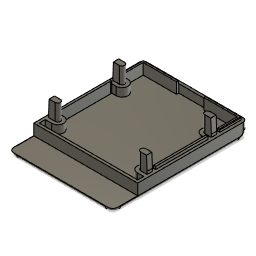
Ensoniq Cartridge Case EEPROM v32 (Autodesk Fusion 360 design; units mm, degrees)
Autodesk Fusion 360 part; units mm, degrees
note: some values were not read from the file. Set by a fixed rule: which face or edge a step refers to.
sketch "Sketch1" plane through (0, 0, 0) normal (0, 1, 0) x (1, 0, 0) in component "PCB"
  line L0 (19.8437, -28.575) -> (-19.8437, -28.575)
  line L1 (-19.8437, -28.575) -> (-19.8437, 28.575)
  line L2 (-19.8437, 28.575) -> (19.8438, 28.575)
  line L3 (19.8438, 28.575) -> (19.8437, -28.575)
  line L4 (19.8437, -28.575) -> (-19.8437, 28.575) construction
  line L5 (-19.8437, -28.575) -> (19.8438, 28.575) construction
  circle A0 centre (-19.8437, 20.32) radius 1.5
  circle A1 centre (-19.8437, -9.525) radius 1.5
  circle A2 centre (19.8438, 20.32) radius 1.5
  circle A3 centre (19.8437, -9.525) radius 1.5
  circle A4 centre (-19.8437, 20.32) radius 1.246
  circle A5 centre (19.8438, 20.32) radius 1.246
  circle A6 centre (19.8437, -9.525) radius 1.246
  circle A7 centre (-19.8437, -9.525) radius 1.246
  dimension "d1" = 57.15
  dimension "d2" = 39.6875
  dimension "d3" = 3
  dimension "d4" = 3
  dimension "d5" = 3
  dimension "d6" = 3
  dimension "d7" = 19.05
  dimension "d8" = 29.845
  dimension "d40" = -0.254
  dimension "d41" = -0.254
  dimension "d42" = -0.254
  dimension "d43" = -0.254
  constraint horizontal L0
  constraint perpendicular L0 L1
  constraint parallel L0 L2
  constraint parallel L1 L3
  constraint coincident L4 origin
  constraint coincident L5 origin
  constraint coincident L1 A0.centre
  constraint coincident L1 A1.centre
  constraint coincident L3 A2.centre
  constraint coincident L3 A3.centre
  constraint horizontal A1.centre A3.centre
  constraint horizontal A0.centre A2.centre
  measures "d1" distance of L0.end L1.end
  measures "d2" distance of L1.end L2.end
  measures "d3" diameter of A0
  measures "d4" diameter of A1
  measures "d5" diameter of A2
  measures "d6" diameter of A3
  measures "d7" distance of L0.end A1.centre
  measures "d8" distance of A0.centre A1.centre
extrude "Extrude1" add sketch "Sketch1" along normal blind 1.6 contours L0 L1 L2 L3 A0 A1 A2 A3 makes body 1 in component "PCB"
sketch "Sketch1 (2)" plane through (0, 0, 0) normal (0, 1, 0) x (1, 0, 0) in component "Back"
  line L0 (19.8438, 18.82) -> (19.8437, -8.025) construction
  arc A0 (19.8437, -8.025) -> (19.8437, -11.025) centre (19.8437, -9.525) ccw construction
  line L1 (19.8437, -11.025) -> (19.8437, -28.575) construction
  line L2 (19.8437, -28.575) -> (-19.8437, -28.575) construction
  line L3 (-19.8437, -28.575) -> (-19.8437, -11.025) construction
  arc A1 (-19.8437, -11.025) -> (-19.8437, -8.025) centre (-19.8437, -9.525) ccw construction
  line L4 (-19.8437, -8.025) -> (-19.8437, 18.82) construction
  arc A2 (-19.8437, 18.82) -> (-19.8437, 21.82) centre (-19.8437, 20.32) ccw construction
  line L5 (-19.8437, 21.82) -> (-19.8438, 28.575) construction
  line L6 (-19.8437, 28.575) -> (19.8438, 28.575) construction
  line L7 (19.8438, 28.575) -> (19.8438, 21.82) construction
  arc A3 (19.8438, 21.82) -> (19.8437, 18.82) centre (19.8438, 20.32) ccw construction
  line L8 (24.13, -16.383) -> (-24.13, -16.383)
  line L9 (-24.13, -16.383) -> (-24.13, 34.417)
  line L10 (-24.13, 34.417) -> (24.13, 34.417)
  line L11 (24.13, 34.417) -> (24.13, -16.383)
  line L12 (24.13, -16.383) -> (-24.13, 34.417) construction
  line L13 (-24.13, -16.383) -> (24.13, 34.417) construction
  line L14 (22.86, 33.147) -> (22.86, -15.113)
  line L15 (22.86, -15.113) -> (-22.86, -15.113)
  line L16 (-22.86, -15.113) -> (-22.86, 33.147)
  line L17 (-22.86, 33.147) -> (22.86, 33.147)
  point P0 (0, 9.017)
  dimension "d11" = 48.26
  dimension "d12" = 50.8
  dimension "d13" = 12.192
  dimension "d14" = 1.27
  constraint horizontal L8
  constraint perpendicular L8 L9
  constraint parallel L8 L10
  constraint parallel L9 L11
  constraint coincident L12 P0
  constraint coincident L13 P0
  constraint vertical origin P0
  measures "d11" distance of L9.end L10.end
  measures "d12" distance of L8.end L9.end
  measures "d13" distance of L2 L8
extrude "Extrude1'" add sketch "Sketch1 (2)" against normal blind 5.08 separate body contours L8 L9 L10 L11 | L14 L15 L16 L17 makes body 2 in component "Back"
sketch "Sketch1 (3)" plane through (0, 0, 0) normal (0, 1, 0) x (1, 0, 0) in component "Front"
  line L0 (-24.13, -16.383) -> (-24.13, 34.417)
  line L1 (24.13, -16.383) -> (-24.13, -16.383)
  line L2 (24.13, 34.417) -> (24.13, -16.383)
  line L3 (-24.13, 34.417) -> (24.13, 34.417)
extrude "Extrude1''" add sketch "Sketch1 (3)" along normal blind 6.604 separate body makes body 3 in component "Front"
sketch "Sketch2" plane through (0, 6.604, 0) normal (0, 1, 0) x (-1, 0, 0) in component "Front"
  line L0 (24.13, -34.417) -> (24.13, 16.383)
  line L1 (24.13, 16.383) -> (-24.13, 16.383)
  line L2 (-24.13, 16.383) -> (-24.13, -34.417)
  line L3 (-24.13, -34.417) -> (24.13, -34.417)
  line L4 (24.13, -34.417) -> (-24.13, -34.417)
  line L5 (-24.13, -34.417) -> (-24.13, 16.383)
  line L6 (-24.13, 16.383) -> (24.13, 16.383)
  line L7 (24.13, 16.383) -> (24.13, -34.417)
  line L8 (24.13, 16.383) -> (-24.13, 16.383)
  line L9 (-24.13, 16.383) -> (-24.13, 27.94)
  line L10 (-24.13, 27.94) -> (24.13, 27.94)
  line L11 (24.13, 27.94) -> (24.13, 16.383)
  dimension "d19" = 11.557
  constraint horizontal L8
  constraint vertical L9
  constraint horizontal L10
  constraint vertical L11
  constraint coincident L0.end L1.start
  measures "d19" distance of L0.end L10.end
extrude "Extrude2" add sketch "Sketch2" along normal blind 5.08 bodies 3 in component "Front"
sketch "Sketch2 (2)" plane through (0, -5.08, 0) normal (0, -1, 0) x (1, 0, 0) in component "Back"
  line L0 (-24.13, -34.417) -> (24.13, -34.417)
  line L1 (24.13, -34.417) -> (24.13, 16.383)
  line L2 (24.13, 16.383) -> (-24.13, 16.383)
  line L3 (-24.13, 16.383) -> (-24.13, -34.417)
  line L4 (-24.13, 27.94) -> (24.13, 27.94)
  line L5 (24.13, 27.94) -> (24.13, -34.417)
  line L6 (24.13, -34.417) -> (-24.13, -34.417)
  line L7 (-24.13, -34.417) -> (-24.13, 27.94)
extrude "Extrude2'" add sketch "Sketch2 (2)" along normal blind 1.905 bodies 2 in component "Back"
extrude "Extrude3" cut sketch "Sketch1 (2)" against normal blind 3.81 contours L14 L15 L16 L17 bodies 2 in component "Back"
sketch "Sketch3" plane through (0, 0, 0) normal (0, -1, 0) x (1, 0, 0) in component "Front"
  line L0 (-24.13, 16.383) -> (-24.13, -34.417)
  line L1 (-24.13, -34.417) -> (24.13, -34.417)
  line L2 (24.13, -34.417) -> (24.13, 16.383)
  line L3 (24.13, 16.383) -> (-24.13, 16.383)
  line L4 (-22.86, 15.113) -> (-22.86, -33.147)
  line L5 (22.86, 15.113) -> (-22.86, 15.113)
  line L6 (22.86, -33.147) -> (22.86, 15.113)
  line L7 (-22.86, -33.147) -> (22.86, -33.147)
extrude "Extrude3'" cut sketch "Sketch1 (2)" along normal blind 8.89 contours L14 L15 L16 L17 bodies 3 in component "Front"
combine "Combine1" operation cut target body 3 tool bodies 1 keep tools in component "Front"
sketch "Sketch3 (2)" plane through (0, -3.81, 0) normal (0, 1, 0) x (-1, 0, 0) in component "Back"
  line L0 (22.86, -33.147) -> (22.86, 15.113)
  line L1 (22.86, 15.113) -> (-22.86, 15.113)
  line L2 (-22.86, 15.113) -> (-22.86, -33.147)
  line L3 (-22.86, -33.147) -> (22.86, -33.147)
  circle A0 centre (-19.8438, -20.32) radius 1.5
  circle A1 centre (19.8437, -20.32) radius 1.5
  circle A2 centre (19.8437, 9.525) radius 1.5
  circle A3 centre (-19.8437, 9.525) radius 1.5
  circle A4 centre (19.8437, -20.32) radius 2.77
  circle A5 centre (-19.8438, -20.32) radius 2.77
  circle A6 centre (19.8437, 9.525) radius 2.77
  circle A7 centre (-19.8437, 9.525) radius 2.77
  line L4 (19.8437, -23.09) -> (22.86, -23.09)
  line L5 (19.8437, -17.55) -> (22.86, -17.55)
  line L6 (-19.8438, -23.09) -> (-22.86, -23.09)
  line L7 (-19.8438, -17.55) -> (-22.86, -17.55)
  line L8 (-19.8437, 6.755) -> (-22.86, 6.755)
  line L9 (-19.8437, 12.295) -> (-22.86, 12.295)
  line L10 (19.8437, 6.755) -> (22.86, 6.755)
  line L11 (19.8437, 12.295) -> (22.86, 12.295)
  circle A8 centre (19.8437, 9.525) radius 1.246
  circle A9 centre (-19.8437, 9.525) radius 1.246
  circle A10 centre (-19.8438, -20.32) radius 1.246
  circle A11 centre (19.8437, -20.32) radius 1.246
  line L12 (19.8437, 8.279) -> (22.86, 8.279)
  line L13 (19.8437, 10.771) -> (22.86, 10.771)
  line L14 (19.8437, -21.566) -> (22.86, -21.566)
  line L15 (19.8437, -19.074) -> (22.86, -19.074)
  line L16 (-19.8438, -21.566) -> (-22.86, -21.566)
  line L17 (-19.8438, -19.074) -> (-22.86, -19.074)
  line L18 (-19.8437, 10.771) -> (-22.86, 10.771)
  line L19 (-19.8437, 8.279) -> (-22.86, 8.279)
  point P0 (19.8437, -20.32)
  point P1 (19.8437, 9.525)
  point P2 (-19.8437, 9.525)
  point P3 (-19.8438, -20.32)
  dimension "d32" = 1.27
  dimension "d33" = 1.27
  dimension "d34" = 1.27
  dimension "d35" = 1.27
  dimension "d44" = -0.254
  dimension "d45" = -0.254
  dimension "d46" = -0.254
  dimension "d47" = -0.254
  constraint coincident A4 L4.start
  constraint coincident L0 L4.end
  constraint tangent A4 L4
  constraint perpendicular L0 L4
  constraint coincident A4 L5.start
  constraint coincident L0 L5.end
  constraint tangent A4 L5
  constraint perpendicular L0 L5
  constraint coincident A5 L6.start
  constraint coincident L2 L6.end
  constraint tangent A5 L6
  constraint perpendicular L2 L6
  constraint coincident A5 L7.start
  constraint coincident L2 L7.end
  constraint tangent A5 L7
  constraint perpendicular L2 L7
  constraint coincident A7 L8.start
  constraint tangent A7 L8
  constraint perpendicular L2 L8
  constraint coincident A7 L9.start
  constraint coincident L2 L9.end
  constraint tangent A7 L9
  constraint perpendicular L2 L9
  constraint coincident A6 L10.start
  constraint tangent A6 L10
  constraint perpendicular L0 L10
  constraint coincident A6 L11.start
  constraint coincident L0 L11.end
  constraint tangent A6 L11
  constraint perpendicular L0 L11
  constraint coincident A8 L12.start
  constraint coincident L0 L12.end
  constraint tangent A8 L12
  constraint perpendicular L0 L12
  constraint coincident A8 L13.start
  constraint tangent A8 L13
  constraint perpendicular L0 L13
  constraint coincident A11 L14.start
  constraint tangent A11 L14
  constraint perpendicular L0 L14
  constraint coincident A11 L15.start
  constraint coincident L0 L15.end
  constraint tangent A11 L15
  constraint perpendicular L0 L15
  constraint coincident A10 L16.start
  constraint tangent A10 L16
  constraint perpendicular L2 L16
  constraint coincident A10 L17.start
  constraint tangent A10 L17
  constraint perpendicular L2 L17
  constraint coincident A9 L18.start
  constraint tangent A9 L18
  constraint perpendicular L2 L18
  constraint coincident A9 L19.start
  constraint coincident L2 L19.end
  constraint tangent A9 L19
  constraint perpendicular L2 L19
extrude "Extrude4" add sketch "Sketch3 (2)" along normal blind 3.81 contours L0 A4 L4 L14 | A1 A4 L14 L15 | L2 A5 L6 L16 | L0 A4 L5 L15 | A0 A5 L16 L17 | A1 A11 L14 L15 | L2 A5 L7 L17 | L0 A6 L10 L12 | A0 A10 L16 L17 | A2 A6 L12 L13 | L2 A7 L8 L19 | L0 A6 L11 L13 | A3 A7 L18 L19 | A2 A8 L12 L13 | L2 A7 L9 L18 | A3 A9 L18 L19 picked at (19.7033, -22.6563) picked at (-19.6476, -22.6531) picked at (19.9123, -21.7302) picked at (-19.786, -21.7311) picked at (19.7033, 7.1887) picked at (-19.6476, 7.1919) picked at (19.9123, 8.1148) picked at (-19.786, 8.1139) bodies 2 in component "Back"
extrude "Extrude5" add 8 faces at (-20.8492, -3.81, 9.9403) (-20.8492, -3.81, -19.9047) (-20.8492, -3.81, 9.9403) (-20.8492, -3.81, -19.9047) (21.8546, -3.81, 9.9403) (21.8546, -3.81, -19.9047) (21.8546, -3.81, 9.9403) (21.8546, -3.81, -19.9047) along direction (0, 1, 0) blind 11.43 on bodies 2 bodies 2 in component "Back"
move_face "OffsetFaces1" offset -0.254 2 faces at (-19.8437, 0.5333, 15.9597) (19.8438, 0.5333, 15.5363) on bodies 3 in component "Front"
move_face "OffsetFaces2" offset -0.254 1 faces at (-6.6992, 1.6, 15.5363) on bodies 3 in component "Front"
sketch "Sketch2 (3)" plane through (0, 8.89, 0) normal (0, -1, 0) x (1, 0, 0)
  line L0 (-22.86, 15.113) -> (-22.86, -33.147)
  line L1 (-22.86, -33.147) -> (22.86, -33.147)
  line L2 (22.86, -33.147) -> (22.86, 15.113)
  line L3 (22.86, 15.113) -> (-22.86, 15.113)
  circle A0 centre (19.8437, 9.525) radius 1.5
  circle A1 centre (-19.8437, 9.525) radius 1.5
  circle A2 centre (-19.8437, -20.32) radius 1.5
  circle A3 centre (19.8438, -20.32) radius 1.5
  line L4 (19.685, 5.715) -> (-19.685, 5.715)
  line L5 (-19.685, 5.715) -> (-19.685, -12.065)
  line L6 (-19.685, -12.065) -> (19.685, -12.065)
  line L7 (19.685, -12.065) -> (19.685, 5.715)
  line L8 (19.685, 5.715) -> (-19.685, -12.065) construction
  line L9 (-19.685, 5.715) -> (19.685, -12.065) construction
  line L10 (0, 15.113) -> (0, -33.147) construction
  point P0 (0, -3.175)
  dimension "d50" = 3.81
  dimension "d51" = 17.78
  dimension "d52" = 39.37
  constraint horizontal L4
  constraint perpendicular L4 L5
  constraint parallel L4 L6
  constraint parallel L5 L7
  constraint coincident L8 P0
  constraint coincident L9 P0
  constraint midpoint L3 L10.start
  constraint midpoint L1 L10.end
  constraint coincident P0 L10
  measures "d50" distance of A1.centre L4
  measures "d51" distance of L4.end L5.end
  measures "d52" distance of L4.start L4.end
extrude "Extrude4'" cut sketch "Sketch2 (3)" against normal blind 1.524 contours L4 L5 L6 L7 bodies 3 in component "Front"
sketch "Sketch5" plane through (0, -3.81, 0) normal (0, 1, 0) x (-1, 0, 0) in component "Back"
  line L0 (22.86, -23.09) -> (19.8437, -23.09)
  arc A0 (19.8437, -17.55) -> (19.8438, -23.09) centre (19.8437, -20.32) ccw
  line L1 (19.8437, -17.55) -> (22.86, -17.55)
  line L2 (22.86, -17.55) -> (22.86, 6.755)
  line L3 (22.86, 6.755) -> (19.8437, 6.755)
  arc A1 (19.8437, 12.295) -> (19.8437, 6.755) centre (19.8437, 9.525) ccw
  line L4 (19.8437, 12.295) -> (22.86, 12.295)
  line L5 (22.86, 12.295) -> (22.86, 15.113)
  line L6 (22.86, 15.113) -> (-22.86, 15.113)
  line L7 (-22.86, 15.113) -> (-22.86, 12.295)
  line L8 (-22.86, 12.295) -> (-19.8437, 12.295)
  arc A2 (-19.8437, 6.755) -> (-19.8438, 12.295) centre (-19.8438, 9.525) ccw
  line L9 (-19.8437, 6.755) -> (-22.86, 6.755)
  line L10 (-22.86, 6.755) -> (-22.86, -17.55)
  line L11 (-22.86, -17.55) -> (-19.8438, -17.55)
  arc A3 (-19.8438, -23.09) -> (-19.8438, -17.55) centre (-19.8438, -20.32) ccw
  line L12 (-19.8438, -23.09) -> (-22.86, -23.09)
  line L13 (-22.86, -23.09) -> (-22.86, -33.147)
  line L14 (-22.86, -33.147) -> (22.86, -33.147)
  line L15 (22.86, -33.147) -> (22.86, -23.09)
  arc A4 (19.8437, -17.042) -> (19.8438, -23.598) centre (19.8437, -20.32) ccw
  line L16 (22.352, -23.598) -> (19.8437, -23.598)
  line L17 (22.352, -32.639) -> (22.352, -23.598)
  line L18 (-22.352, -32.639) -> (22.352, -32.639)
  line L19 (-22.352, -23.598) -> (-22.352, -32.639)
  line L20 (-19.8438, -23.598) -> (-22.352, -23.598)
  arc A5 (-19.8438, -23.598) -> (-19.8438, -17.042) centre (-19.8438, -20.32) ccw
  line L21 (-22.352, -17.042) -> (-19.8438, -17.042)
  line L22 (-22.352, 6.247) -> (-22.352, -17.042)
  line L23 (-19.8437, 6.247) -> (-22.352, 6.247)
  arc A6 (-19.8437, 6.247) -> (-19.8438, 12.803) centre (-19.8438, 9.525) ccw
  line L24 (-22.352, 12.803) -> (-19.8438, 12.803)
  line L25 (-22.352, 14.605) -> (-22.352, 12.803)
  line L26 (22.352, 14.605) -> (-22.352, 14.605)
  line L27 (22.352, 12.803) -> (22.352, 14.605)
  line L28 (19.8437, 12.803) -> (22.352, 12.803)
  arc A7 (19.8437, 12.803) -> (19.8437, 6.247) centre (19.8437, 9.525) ccw
  line L29 (22.352, 6.247) -> (19.8437, 6.247)
  line L30 (22.352, -17.042) -> (22.352, 6.247)
  line L31 (19.8437, -17.042) -> (22.352, -17.042)
  line L32 (22.352, 14.605) -> (22.352, 15.113)
  line L33 (-22.352, 14.605) -> (-22.352, 15.113)
  line L34 (-22.352, -23.598) -> (-22.352, -17.042)
  line L35 (-22.352, 6.247) -> (-22.352, 12.803)
  line L36 (22.352, -23.598) -> (22.352, -17.042)
  line L37 (22.352, 6.247) -> (22.352, 12.803)
  line L38 (22.86, -23.368) -> (22.86, -17.55)
  line L39 (-22.86, -23.09) -> (-22.86, -17.55)
  line L40 (-22.86, 6.755) -> (-22.86, 12.295)
  line L41 (22.86, 6.755) -> (22.86, 12.295)
  line L42 (0, -32.639) -> (0, -33.147) construction
  line L43 (6.35, -32.639) -> (6.35, -33.147)
  line L44 (-6.35, -32.639) -> (-6.35, -33.147)
  dimension "d60" = -0.508
  dimension "d70" = 6.35
  dimension "d71" = 6.35
  constraint coincident L6 L32.end
  constraint perpendicular L6 L32
  constraint coincident L6 L33.end
  constraint perpendicular L6 L33
  constraint coincident L1.end L2.start
  constraint coincident L12.end L13.start
  constraint coincident L10.end L11.start
  constraint coincident L9.end L10.start
  constraint coincident L7.end L8.start
  constraint coincident L2.end L3.start
  constraint coincident L4.end L5.start
  constraint midpoint L18 L42.start
  constraint midpoint L14 L42.end
  constraint coincident L18 L43.start
  constraint coincident L14 L43.end
  constraint perpendicular L18 L43
  constraint coincident L18 L44.start
  constraint coincident L14 L44.end
  constraint perpendicular L14 L44
  measures "d70" distance of L42 L43
  measures "d71" distance of L42 L44
extrude "Extrude7" add sketch "Sketch5" along normal blind 5.08 contours L0 L14 L15 L17 L18 L36 L38 L43 | L1 L2 L3 L30 L36 L37 | L12 L13 L14 L18 L19 L34 L44 | L9 L10 L11 L22 L34 L35 bodies 2 in component "Back"
chamfer "Chamfer2" distance 0.254 distance2 0.762 5 edges at (-22.86, 1.27, -28.2575) (-22.86, 1.27, -23.229) (-14.605, 1.27, -33.147) (14.605, 1.27, -33.147) (22.86, 1.27, -28.1185) measured on face at (-17.1873, 1.27, -32.9777) measured on face at (-17.1873, 1.27, -32.9777) measured on face at (-17.1873, 1.27, -32.9777) measured on face at (17.1873, 1.27, -32.9777) measured on face at (17.1873, 1.27, -32.9777) on bodies 2 in component "Back"
chamfer "Chamfer1" distance 0.254 distance2 6.35 4 edges at (-22.86, 7.62, -20.32) (-22.86, 7.62, 9.525) (22.86, 7.62, -20.32) (22.86, 7.62, 9.525) measured on face at (-20.8492, 7.62, -19.9047) measured on face at (-20.8492, 7.62, 9.9403) measured on face at (21.8546, 7.62, -19.9047) measured on face at (21.8546, 7.62, 9.9403) on bodies 2 in component "Back"
move_face "OffsetFaces1'" offset -0.127 5 faces at (-22.86, 0.3387, -29.8873) (-22.86, 0.1693, -23.2753) (-11.8533, 0.3387, -33.147) (17.3567, 0.1693, -33.147) (22.86, 0.3387, -29.7947) on bodies 2 in component "Back"
sketch "Sketch6" plane through (0, 0, 16.383) normal (0, 0, 1) x (1, 0, 0) in component "Back"
  line L0 (24.13, 0) -> (-24.13, 0)
  line L1 (-24.13, 0) -> (-24.13, -5.08)
  line L2 (-24.13, -5.08) -> (24.13, -5.08)
  line L3 (24.13, -5.08) -> (24.13, 0)
extrude "Extrude8" add sketch "Sketch6" along normal blind 11.557 bodies 2 in component "Back"
fillet "Fillet1" chord length 2.54 8 edges at (0, -6.985, 27.94) (24.13, -6.985, -3.2385) (24.13, -3.4925, -34.417) (0, -6.985, -34.417) (-24.13, -6.985, -3.2385) (-24.13, -3.4925, -34.417) (-24.13, -3.4925, 27.94) (24.13, -3.4925, 27.94) on bodies 2 in component "Back"
extrude "Extrude9" cut sketch "Sketch6" along normal blind 16.002 bodies 2 in component "Back"
sketch "Sketch5 (2)" plane through (0, 8.89, 0) normal (0, -1, 0) x (1, 0, 0) in component "Front"
  line L0 (-19.685, 5.715) -> (19.685, 5.715)
  line L1 (19.685, 5.715) -> (19.685, -12.065)
  line L2 (19.685, -12.065) -> (-19.685, -12.065)
  line L3 (-19.685, -12.065) -> (-19.685, 5.715)
  line L4 (-22.86, 15.113) -> (-22.86, -33.147)
  line L5 (-22.86, -33.147) -> (22.86, -33.147)
  line L6 (22.86, -33.147) -> (22.86, 15.113)
  line L7 (22.86, 15.113) -> (-22.86, 15.113)
  line L8 (-6.35, -32.639) -> (-6.35, -33.147)
  line L9 (22.352, -32.639) -> (-22.352, -32.639)
  line L10 (6.35, -32.639) -> (6.35, -33.147)
  line L11 (22.86, -33.147) -> (-22.86, -33.147)
extrude "Extrude6" add sketch "Sketch5 (2)" along normal blind 10.16 contours L5 L8 L9 L10 L11 bodies 3 in component "Front"
chamfer "Chamfer1'" distance 0.254 distance2 0.762 1 edges at (0, -1.27, -33.147) measured on face at (-2.1167, -1.27, -32.9777) on bodies 3 in component "Front"
move_face "OffsetFaces3" offset -0.127 1 faces at (-2.1167, -0.1693, -33.147) on bodies 3 in component "Front"
fillet "Fillet1'" chord length 2.54 8 edges at (24.13, 9.144, 27.94) (0, 11.684, 27.94) (24.13, 11.684, -3.2385) (-24.13, 11.684, -3.2385) (-24.13, 9.144, 27.94) (24.13, 5.842, -34.417) (0, 11.684, -34.417) (-24.13, 5.842, -34.417) on bodies 3 in component "Front"
sketch "Sketch4" plane through (0, 6.604, 0) normal (0, -1, 0) x (1, 0, 0) in component "Front"
  line L0 (-24.13, 26.1439) -> (-24.13, 16.383)
  line L1 (-24.13, 16.383) -> (24.13, 16.383)
  line L2 (24.13, 16.383) -> (24.13, 26.1439)
  line L3 (22.3339, 27.94) -> (-22.3339, 27.94)
  line L4 (-22.86, 17.653) -> (-22.86, 16.383)
  line L5 (22.86, 17.653) -> (22.86, 16.383)
  line L6 (22.86, 17.653) -> (22.86, 26.1439)
  spline S0 degree 3 poles (22.3339, 26.67) (22.4034, 26.67) (22.4722, 26.6562) (22.5363, 26.6295) (22.6012, 26.6025) (22.66, 26.5627) (22.7093, 26.5125) (22.7566, 26.4643) (22.7943, 26.4074) (22.8201, 26.345) (22.8464, 26.2812) (22.86, 26.2129) (22.86, 26.1439) knots 0 0 0 0 0.071145 0.071145 0.071145 0.143155 0.143155 0.143155 0.212385 0.212385 0.212385 0.283027 0.283027 0.283027 0.283027
  line L7 (22.3339, 26.67) -> (-22.3339, 26.67)
  spline S1 degree 3 poles (-22.86, 26.1439) (-22.86, 26.2134) (-22.8462, 26.2822) (-22.8195, 26.3463) (-22.7925, 26.4112) (-22.7527, 26.47) (-22.7025, 26.5193) (-22.6543, 26.5666) (-22.5974, 26.6043) (-22.535, 26.6301) (-22.4712, 26.6564) (-22.4029, 26.67) (-22.3339, 26.67) knots 0 0 0 0 0.071145 0.071145 0.071145 0.143155 0.143155 0.143155 0.212385 0.212385 0.212385 0.283027 0.283027 0.283027 0.283027
  line L8 (-22.86, 26.1439) -> (-22.86, 17.653)
  line L9 (-22.86, 17.653) -> (22.86, 17.653)
  spline S2 degree 3 poles (-24.13, 26.1439) (-24.13, 26.3811) (-24.083, 26.6159) (-23.8995, 27.0564) (-23.7637, 27.2572) (-23.4278, 27.5871) (-23.2335, 27.7155) (-22.8026, 27.8937) (-22.5694, 27.94) (-22.3339, 27.94) knots 0 0 0 0 0.071145 0.071145 0.143155 0.143155 0.212385 0.212385 0.283027 0.283027 0.283027 0.283027
  spline S3 degree 3 poles (22.3339, 27.94) (22.5711, 27.94) (22.8059, 27.893) (23.2464, 27.7095) (23.4472, 27.5737) (23.7771, 27.2378) (23.9055, 27.0435) (24.0837, 26.6126) (24.13, 26.3794) (24.13, 26.1439) knots 0 0 0 0 0.071145 0.071145 0.143155 0.143155 0.212385 0.212385 0.283027 0.283027 0.283027 0.283027
  constraint coincident L1 L4.end
  constraint perpendicular L1 L4
  constraint coincident L1 L5.end
  constraint perpendicular L1 L5
  constraint parallel L2 L6
  constraint parallel L3 L7
  constraint parallel L0 L8
  constraint parallel L1 L9
extrude "Extrude5'" cut sketch "Sketch4" against normal blind 3.81 contours L1 L4 L5 L9 | L6 S0 L7 S1 L8 L9 bodies 3 in component "Front"
move_face "OffsetFaces2'" offset 0.508 12 faces at (-22.352, -0.8467, 6.4163) (-22.352, -0.8467, 2.7032) (-22.352, -2.54, -17.3807) (-22.352, -0.8467, -23.4287) (-22.352, -0.4233, -26.6117) (-17.018, -2.1167, -32.639) (11.684, -2.1167, -32.639) (22.352, -0.4233, -29.6253) (22.352, -0.8467, -23.4287) (22.352, -2.54, -17.3807) (22.352, -0.8467, 2.7032) (22.352, -0.8467, 6.4163) on bodies 2 in component "Back"
move_face "OffsetFaces5" offset 0.508 1 faces at (2.1167, 5.5033, -32.639) on bodies 3 in component "Front"
move_body "Move2" bodies 3 to x (1, 0, 0) y (0, 1, 0) z (0, 0, 1) at (0, 13.97, 0) in component "Front"
component "PCB" placed x (1, 0, 0) y (0, 1, 0) z (0, 0, 1) at (0, 0, 0)
component "Back" placed x (1, 0, 0) y (0, 1, 0) z (0, 0, 1) at (0, 0, 0)
component "Front" placed x (1, 0, 0) y (0, 1, 0) z (0, 0, 1) at (0, 0, 0)
